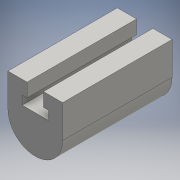
# Autodesk Inventor part: BallBallerina_StopHead
Saved by Autodesk Inventor 2016 (Build 200138000, 138)
## iProperties
Created: 2016-04-11
Part Number: BallBallerina_StopHead
Material: Generic
Document SubType Name: Modeling
Designer: Admin
Density: 1 g/cm^3
Appearance: Default
Author: Admin
Autodesk Inventor part; units mm, degrees
ref_plane "YZ Plane" through (0, 0, 0) normal (1, 0, 0) x (0, 1, 0)
ref_plane "XZ Plane" through (0, 0, 0) normal (0, 1, 0) x (-1, 0, 0)
ref_plane "XY Plane" through (0, 0, 0) normal (0, 0, 1) x (1, 0, 0)
sketch "Sketch1" plane through (0, 0, 0) normal (0, 1, 0) x (-1, 0, 0)
  line L0 (7, 0) -> (-7, 0) projected
  line L1 (0, -13.2) -> (0, 2.2) projected
  line L2 (-5, 0) -> (-5, -6)
  line L3 (5, -6) -> (5, 0)
  line L4 (1.5, 0) -> (1.5, -2.5)
  line L5 (1.5, -2.5) -> (2.3876, -2.5)
  line L6 (2.3876, -2.5) -> (2.3876, -4.1002)
  line L7 (2.3876, -4.1002) -> (0, -4.1002)
  line L8 (-1.5, 0) -> (-1.5, -2.5)
  line L9 (-1.5, -2.5) -> (-2.3876, -2.5)
  line L10 (-2.3876, -2.5) -> (-2.3876, -4.1002)
  line L11 (-2.3876, -4.1002) -> (0, -4.1002)
  line L12 (5, 0) -> (1.5, 0)
  line L13 (-1.5, 0) -> (-5, 0)
  arc A0 (-5, -6) -> (5, -6) centre (0, -6) ccw
  point P0 (0, 0)
  dimension "d0" = 10
  dimension "d1" = 5
  dimension "d3" = 2.3876
  dimension "d4" = 1.6002
  dimension "d5" = 2.5
  dimension "d6" = 1.5
  dimension "d7" = 6
  dimension "d8" = 5
  constraints: 24 end point, 5 perpendicular, 4 point on line, 4 symmetric about line, 2 horizontal, 2 point on circle, 1 centre point, 1 parallel, 1 vertical
  measures "d0" distance of L2.end L3.start
  measures "d1" distance between parallel lines of L1 L3
  measures "d3" distance of L6.end L7.end
  measures "d4" distance of L5.end L6.end
  measures "d5" distance of L4.start L4.end
  measures "d6" distance between parallel lines of L1 L4
  measures "d7" distance of L2.start L2.end
  measures "d8" distance between parallel lines of L1 L2
extrude "Extrusion1" add sketch "Sketch1" along normal blind 20 contours L3 A0 L1 L7 L6 L5 L4 L0 | A0 L2 L0 L8 L9 L10 L11 L1
sketch "Sketch2" plane through (-2.3876, 0, -4.1002) normal (0, 0, 1) x (1, 0, 0)
  line L0 (2.3876, 0) -> (2.3876, 20) construction
  line L1 (7.3876, 20) -> (-2.6124, 20) projected
  circle A0 centre (2.3876, 10) radius 1.5
  dimension "d11" = 3
  constraints: 2 end point, 2 midpoint, 1 centre point
  measures "d11" diameter of A0
extrude "Extrusion2" cut sketch "Sketch2" against normal blind 20
equation "\"d1\" = 0.5 * d0"
body "Solid1"
